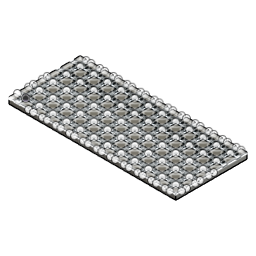
Holder Parametrico V1 (Autodesk Fusion 360 design; units mm, degrees)
Autodesk Fusion 360 part; units mm, degrees
sketch "Boceto1" plane through (0, 0, 0) normal (0, 1, 0) x (1, 0, 0)
  circle A0 centre (0, 0) radius 10.5
  line L0 (0, 0) -> (-13.5, 0)
  line L1 (-13.5, 0) -> (-13.5, -13.5)
  line L2 (-13.5, -13.5) -> (257.7, -13.5)
  line L3 (257.7, -13.5) -> (257.7, 102.3)
  line L4 (257.7, 102.3) -> (-13.5, 102.3)
  line L5 (-13.5, 102.3) -> (-13.5, -13.5)
  line L6 (0, 0) -> (0, -13.5)
  line L7 (-13.5, 0) -> (-13.5, 4)
  line L8 (-13.5, 4) -> (-13.5, -4)
  line L9 (0, -13.5) -> (-4, -13.5)
  line L10 (-4, -13.5) -> (4, -13.5)
  line L11 (-4, -13.5) -> (-4, 102.3)
  line L12 (4, -13.5) -> (4, 102.3)
  line L13 (-13.5, 4) -> (257.7, 4)
  line L14 (-13.5, -4) -> (257.7, -4)
  line L15 (-13.5, 18.2) -> (257.7, 18.2)
  line L16 (-13.5, 26.2) -> (257.7, 26.2)
  line L17 (-13.5, 40.4) -> (257.7, 40.4)
  line L18 (-13.5, 48.4) -> (257.7, 48.4)
  line L19 (-13.5, -13.5) -> (-10.5, -13.5)
  line L20 (-10.5, -13.5) -> (-10.5, -10.5)
  line L21 (-10.5, -10.5) -> (-13.5, -10.5)
  line L22 (-13.5, -10.5) -> (-13.5, -13.5)
  line L23 (-10.5, -10.5) -> (254.7, -10.5)
  line L24 (254.7, -10.5) -> (254.7, 99.3)
  line L25 (254.7, 99.3) -> (-10.5, 99.3)
  line L26 (-10.5, 99.3) -> (-10.5, -10.5)
  line L27 (-13.5, -13.5) -> (-11.5, -13.5)
  line L28 (-11.5, -13.5) -> (-11.5, -11.5)
  line L29 (-11.5, -11.5) -> (-13.5, -11.5)
  line L30 (-13.5, -11.5) -> (-13.5, -13.5)
  line L31 (-11.5, -11.5) -> (255.7, -11.5)
  line L32 (255.7, -11.5) -> (255.7, 100.3)
  line L33 (255.7, 100.3) -> (-11.5, 100.3)
  line L34 (-11.5, 100.3) -> (-11.5, -11.5)
  line L35 (0, 0) -> (-13.5, 0)
  circle A1 centre (22.2, 0) radius 10.5
  line L36 (18.2, -13.5) -> (18.2, 102.3)
  line L37 (26.2, -13.5) -> (26.2, 102.3)
  circle A2 centre (0, 22.2) radius 10.5
  circle A3 centre (22.2, 22.2) radius 10.5
  circle A4 centre (44.4, 0) radius 10.5
  circle A5 centre (44.4, 22.2) radius 10.5
  line L38 (40.4, -13.5) -> (40.4, 102.3)
  line L39 (48.4, -13.5) -> (48.4, 102.3)
  circle A6 centre (0, 44.4) radius 10.5
  circle A7 centre (22.2, 44.4) radius 10.5
  circle A8 centre (44.4, 44.4) radius 10.5
  circle A9 centre (66.6, 0) radius 10.5
  circle A10 centre (88.8, 0) radius 10.5
  circle A11 centre (111, 0) radius 10.5
  circle A12 centre (133.2, 0) radius 10.5
  circle A13 centre (66.6, 22.2) radius 10.5
  circle A14 centre (88.8, 22.2) radius 10.5
  circle A15 centre (111, 22.2) radius 10.5
  circle A16 centre (133.2, 22.2) radius 10.5
  circle A17 centre (66.6, 44.4) radius 10.5
  circle A18 centre (88.8, 44.4) radius 10.5
  circle A19 centre (111, 44.4) radius 10.5
  circle A20 centre (133.2, 44.4) radius 10.5
  line L40 (62.6, -13.5) -> (62.6, 102.3)
  line L41 (70.6, -13.5) -> (70.6, 102.3)
  line L42 (84.8, -13.5) -> (84.8, 102.3)
  line L43 (92.8, -13.5) -> (92.8, 102.3)
  line L44 (107, -13.5) -> (107, 102.3)
  line L45 (115, -13.5) -> (115, 102.3)
  line L46 (129.2, -13.5) -> (129.2, 102.3)
  line L47 (137.2, -13.5) -> (137.2, 102.3)
  circle A21 centre (0, 66.6) radius 10.5
  circle A22 centre (22.2, 66.6) radius 10.5
  circle A23 centre (44.4, 66.6) radius 10.5
  circle A24 centre (66.6, 66.6) radius 10.5
  circle A25 centre (88.8, 66.6) radius 10.5
  circle A26 centre (111, 66.6) radius 10.5
  circle A27 centre (133.2, 66.6) radius 10.5
  circle A28 centre (0, 88.8) radius 10.5
  circle A29 centre (22.2, 88.8) radius 10.5
  circle A30 centre (44.4, 88.8) radius 10.5
  circle A31 centre (66.6, 88.8) radius 10.5
  circle A32 centre (88.8, 88.8) radius 10.5
  circle A33 centre (111, 88.8) radius 10.5
  circle A34 centre (133.2, 88.8) radius 10.5
  circle A35 centre (155.4, 0) radius 10.5
  circle A36 centre (177.6, 0) radius 10.5
  circle A37 centre (199.8, 0) radius 10.5
  circle A38 centre (155.4, 22.2) radius 10.5
  circle A39 centre (177.6, 22.2) radius 10.5
  circle A40 centre (199.8, 22.2) radius 10.5
  circle A41 centre (155.4, 44.4) radius 10.5
  circle A42 centre (177.6, 44.4) radius 10.5
  circle A43 centre (199.8, 44.4) radius 10.5
  circle A44 centre (155.4, 66.6) radius 10.5
  circle A45 centre (177.6, 66.6) radius 10.5
  circle A46 centre (199.8, 66.6) radius 10.5
  circle A47 centre (155.4, 88.8) radius 10.5
  circle A48 centre (177.6, 88.8) radius 10.5
  circle A49 centre (199.8, 88.8) radius 10.5
  line L48 (151.4, -13.5) -> (151.4, 102.3)
  line L49 (159.4, -13.5) -> (159.4, 102.3)
  line L50 (173.6, -13.5) -> (173.6, 102.3)
  line L51 (181.6, -13.5) -> (181.6, 102.3)
  line L52 (195.8, -13.5) -> (195.8, 102.3)
  line L53 (203.8, -13.5) -> (203.8, 102.3)
  circle A50 centre (222, 0) radius 10.5
  circle A51 centre (244.2, 0) radius 10.5
  circle A52 centre (222, 22.2) radius 10.5
  circle A53 centre (244.2, 22.2) radius 10.5
  circle A54 centre (222, 44.4) radius 10.5
  circle A55 centre (244.2, 44.4) radius 10.5
  circle A56 centre (222, 66.6) radius 10.5
  circle A57 centre (244.2, 66.6) radius 10.5
  circle A58 centre (222, 88.8) radius 10.5
  circle A59 centre (244.2, 88.8) radius 10.5
  line L54 (218, -13.5) -> (218, 102.3)
  line L55 (226, -13.5) -> (226, 102.3)
  line L56 (240.2, -13.5) -> (240.2, 102.3)
  line L57 (248.2, -13.5) -> (248.2, 102.3)
  dimension "d7" = 21
  dimension "d10" = 22.2
  dimension "d11" = 22.2
  dimension "d12" = 13.5
  dimension "d13" = 13.5
  dimension "d14" = 271.2
  dimension "d15" = 115.8
  dimension "d16" = 13.5
  dimension "d17" = 4
  dimension "d18" = 8
  dimension "d19" = 4
  dimension "d20" = 8
  dimension "d21" = 115.8
  dimension "d22" = 115.8
  dimension "d23" = 271.2
  dimension "d24" = 271.2
  dimension "d27" = 22.2
  dimension "d28" = 0
  dimension "d31" = 0
  dimension "d32" = 22.2
  dimension "d33" = 3
  dimension "d34" = 3
  dimension "d35" = 265.2
  dimension "d36" = 109.8
  dimension "d37" = 2
  dimension "d38" = 2
  dimension "d39" = 267.2
  dimension "d40" = 111.8
  dimension "EspaciaxoExtra1" = 13.5
  constraint coincident A0.centre L0.start
  constraint horizontal L0
  constraint perpendicular L0 L1
  constraint horizontal L2
  constraint vertical L3
  constraint horizontal L4
  constraint vertical L5
  constraint perpendicular L2 L6
  constraint perpendicular L0 L7
  constraint perpendicular L0 L8
  constraint perpendicular L6 L9
  constraint perpendicular L6 L10
  constraint perpendicular L9 L11
  constraint perpendicular L10 L12
  constraint perpendicular L12 L13
  constraint perpendicular L12 L14
  constraint horizontal L19
  constraint vertical L20
  constraint horizontal L21
  constraint vertical L22
  constraint horizontal L23
  constraint vertical L24
  constraint horizontal L25
  constraint vertical L26
  constraint horizontal L27
  constraint vertical L28
  constraint horizontal L29
  constraint vertical L30
  constraint horizontal L31
  constraint vertical L32
  constraint horizontal L33
  constraint vertical L34
  constraint perpendicular L1 L35
  measures "d7" diameter of A0
  measures "d12" distance of A0.centre L0.end
  measures "d13" distance of L0.end L1.end
  measures "d14" distance of L1.end L2.end
  measures "d15" distance of L1.end L4.end
  measures "d16" distance of A0.centre L6.end
  measures "d17" distance of L0.end L7.end
  measures "d18" distance of L7.end L8.end
  measures "d19" distance of L6.end L9.end
  measures "d20" distance of L9.end L10.end
  measures "d21" distance of L9.end L11.end
  measures "d22" distance of L10.end L12.end
  measures "d23" distance of L7.end L13.end
  measures "d24" distance of L8.end L14.end
  measures "d33" distance of L1.end L19.end
  measures "d34" distance of L1.end L21.end
  measures "d35" distance of L20.end L23.end
  measures "d36" distance of L20.end L25.end
  measures "d37" distance of L1.end L27.end
  measures "d38" distance of L1.end L29.end
  measures "d39" distance of L28.end L31.end
  measures "d40" distance of L28.end L33.end
  measures "EspaciaxoExtra1" distance of A0.centre L0.end
extrude "Extruir1" add sketch "Boceto1" against normal blind 8
sketch "Boceto2" plane through (0, 0, 0) normal (0, 1, 0) x (1, 0, 0)
  circle A0 centre (0, 0) radius 10.5
  dimension "d43" = 21
  constraint coincident A0.centre origin
  measures "d43" diameter of A0
extrude "Extruir4" cut sketch "Boceto2" against normal up to surface (8 mm away)
pattern_linear "Patrón R1" count 12 spacing 22.2 along (1, 0, 0) count 5 spacing 22.2 along (0, 0, -1) of "Extruir4"
extrude "Extruir6" add sketch "Boceto1" along normal blind 2 contours A0 L11 L14 L23 L26 | A0 L11 L14 | L11 L20 L23 L31 | L2 L11 L20 L31 | L20 L21 L31 L34 | L14 L21 L26 L34 | L2 L19 L20 L28 L31 | L1 L5 L21 L22 L29 L34 | L1 L5 L14 L21 L34 | L1 L2 L5 L19 L22 L27 L28 L29 L30
pattern_linear "Patrón R7" count 2 spacing 261.7 along (1, 0, 0) count 2 spacing 106.3 along (0, 0, -1) of "Extruir6"
extrude "Extruir7" add sketch "Boceto1" along normal blind 2 contours A0 L11 L13 | A0 L11 L13 L15 L26 A2 | L11 L15 A2 | L13 L15 L26 L34 | L5 L13 L15 L34
pattern_linear "Patrón R3" count 4 spacing 22.2 along (0, 0, -1) count 2 spacing 261.7 along (1, 0, 0) of "Extruir7"
extrude "Extruir8" add sketch "Boceto1" along normal blind 2 contours A0 L12 L14 L23 A1 L36 | A0 L12 L14 | L14 A1 L36 | L12 L23 L31 L36 | L2 L12 L31 L36
pattern_linear "Patrón R8" count 11 spacing 22.2 along (1, 0, 0) count 2 spacing 106.3 along (0, 0, -1) of "Extruir8"
extrude "Extruir5" add sketch "Boceto1" along normal blind 2 contours A0 L12 L13 | A0 L12 L13 L15 A1 L36 A2 A3 | L13 A1 L36 | L12 L15 A2 | L15 L36 A3
pattern_linear "Patrón R2" count 11 spacing 22.2 along (1, 0, 0) count 4 spacing 22.2 along (0, 0, -1) of "Extruir5"
equation "DiametroCeldas = 21 mm"
equation "EspaciadoEntreCeldas = 1.2 mm" comment "para 2 perimetros 1.2mm, ara 4 perimetros 2mm"
equation "AnchoNiquel = 8 mm"
equation "AlturaAireNiquel = 2 mm"
equation "MargenPerimetral = 3 mm"
equation "AlturaPerimetral = AnchoNiquel"
equation "d7 = DiametroCeldas"
equation "Series = 12"
equation "Paralelos = 5"
equation "d10 = DiametroCeldas + EspaciadoEntreCeldas"
equation "d11 = DiametroCeldas + EspaciadoEntreCeldas"
equation "d12 = ( DiametroCeldas / 2 ) + MargenPerimetral"
equation "d13 = ( DiametroCeldas / 2 ) + MargenPerimetral"
equation "d14 = ( MargenPerimetral * 2 ) + ( DiametroCeldas * Series ) + ( EspaciadoEntreCeldas * Series ) - EspaciadoEntreCeldas"
equation "d15 = ( MargenPerimetral * 2 ) + ( DiametroCeldas * Paralelos ) + ( EspaciadoEntreCeldas * Paralelos ) - EspaciadoEntreCeldas"
equation "d16 = ( DiametroCeldas / 2 ) + MargenPerimetral"
equation "d17 = AnchoNiquel / 2"
equation "d18 = AnchoNiquel"
equation "d19 = AnchoNiquel / 2"
equation "d20 = AnchoNiquel"
equation "d21 = ( MargenPerimetral * 2 ) + ( DiametroCeldas * Paralelos ) + ( EspaciadoEntreCeldas * Paralelos ) - EspaciadoEntreCeldas"
equation "d22 = ( MargenPerimetral * 2 ) + ( DiametroCeldas * Paralelos ) + ( EspaciadoEntreCeldas * Paralelos ) - EspaciadoEntreCeldas"
equation "d23 = ( MargenPerimetral * 2 ) + ( DiametroCeldas * Series ) + ( EspaciadoEntreCeldas * Series ) - EspaciadoEntreCeldas"
equation "d24 = ( MargenPerimetral * 2 ) + ( DiametroCeldas * Series ) + ( EspaciadoEntreCeldas * Series ) - EspaciadoEntreCeldas"
equation "d25 = Series"
equation "d27 = ( DiametroCeldas / 2 ) + ( DiametroCeldas / 2 ) + EspaciadoEntreCeldas"
equation "d32 = ( DiametroCeldas / 2 ) + ( DiametroCeldas / 2 ) + EspaciadoEntreCeldas"
equation "d33 = MargenPerimetral"
equation "d34 = MargenPerimetral"
equation "d35 = ( MargenPerimetral ) + ( DiametroCeldas * Series ) + ( EspaciadoEntreCeldas * Series ) - ( MargenPerimetral ) - EspaciadoEntreCeldas"
equation "d36 = ( DiametroCeldas * Paralelos ) + ( ( EspaciadoEntreCeldas * Paralelos ) - EspaciadoEntreCeldas )"
equation "d37 = AlturaAireNiquel"
equation "d38 = AlturaAireNiquel"
equation "d39 = ( ( MargenPerimetral * 2 ) + ( DiametroCeldas * Series ) + ( EspaciadoEntreCeldas * Series ) - EspaciadoEntreCeldas ) - ( AlturaAireNiquel * 2 )"
equation "d40 = ( ( MargenPerimetral * 2 ) + ( DiametroCeldas * Paralelos ) + ( EspaciadoEntreCeldas * Paralelos ) - EspaciadoEntreCeldas ) - ( AlturaAireNiquel * 2 )"
equation "d41 = -AlturaPerimetral"
equation "d43 = DiametroCeldas"
equation "d50 = Series"
equation "d51 = Paralelos"
equation "d52 = EspaciadoEntreCeldas + DiametroCeldas"
equation "d53 = DiametroCeldas + EspaciadoEntreCeldas"
equation "d54 = AlturaAireNiquel"
equation "d56 = Series - 1"
equation "d57 = Paralelos - 1"
equation "d58 = DiametroCeldas + EspaciadoEntreCeldas"
equation "d59 = DiametroCeldas + EspaciadoEntreCeldas"
equation "d60 = AlturaAireNiquel"
equation "d62 = AlturaAireNiquel"
equation "d64 = AlturaAireNiquel"
equation "d66 = Paralelos - 1"
equation "d68 = ( DiametroCeldas + EspaciadoEntreCeldas - AnchoNiquel ) + AnchoNiquel"
equation "d69 = ( MargenPerimetral + DiametroCeldas * Series ) + ( ( EspaciadoEntreCeldas * Series ) - EspaciadoEntreCeldas ) - ( EspaciaxoExtra1 - MargenPerimetral - ( AnchoNiquel / 2 ) )"
equation "EspaciaxoExtra1 = ( DiametroCeldas / 2 ) + MargenPerimetral"
equation "d85 = ( MargenPerimetral + DiametroCeldas * Series ) + ( ( EspaciadoEntreCeldas * Series ) - EspaciadoEntreCeldas ) - ( EspaciaxoExtra1 - MargenPerimetral - ( AnchoNiquel / 2 ) )"
equation "d86 = -( ( MargenPerimetral + DiametroCeldas * Paralelos ) + ( ( EspaciadoEntreCeldas * Paralelos ) - EspaciadoEntreCeldas ) - ( EspaciaxoExtra1 - MargenPerimetral - ( AnchoNiquel / 2 ) ) )"
equation "d87 = Series - 1"
equation "d89 = DiametroCeldas + EspaciadoEntreCeldas"
equation "d90 = -( ( MargenPerimetral + DiametroCeldas * Paralelos ) + ( ( EspaciadoEntreCeldas * Paralelos ) - EspaciadoEntreCeldas ) - ( EspaciaxoExtra1 - MargenPerimetral - ( AnchoNiquel / 2 ) ) )"
